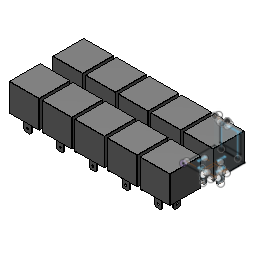
Блок реле с прозрачной крышкой т2 v2 (Autodesk Fusion 360 design; units mm, degrees)
Autodesk Fusion 360 part; units mm, degrees
sketch "Sketch1" plane through (0, 0, 0) normal (0, 0, 1) x (1, 0, 0)
  line L0 (0, 0) -> (27.5, 0)
  line L1 (27.5, 0) -> (27.5, 28.5)
  line L2 (27.5, 28.5) -> (0, 28.5)
  line L3 (0, 28.5) -> (0, 0)
  dimension "d1" = 27.5
  dimension "d2" = 28.5
  constraint horizontal L0
  constraint vertical L1
  constraint horizontal L2
  constraint vertical L3
  constraint coincident L0.start L3.end
  measures "d1" distance of L0.start L0.end
  measures "d2" distance of L0.start L2.end
extrude "Extrude1" add sketch "Sketch1" along normal blind 25.2 makes body 1
sketch "Sketch2" plane through (0, 0, 0) normal (0, 0, 1) x (1, 0, 0)
  line L0 (0, 3) -> (17, 3) construction
  line L1 (27.5, 4) -> (10.5, 4) construction
  line L2 (18, 0) -> (18, 4) construction
  line L3 (17, 4) -> (10.5, 4)
  line L4 (10.5, 4) -> (10.5, 3.1)
  line L5 (10.5, 3.1) -> (17, 3.1)
  line L6 (17, 3.1) -> (17, 4)
  line L7 (25, 0) -> (25, 15) construction
  line L8 (25, 15) -> (24, 15) construction
  line L9 (24, 15) -> (24, 8.7) construction
  line L10 (27.5, 12) -> (21.5, 12) construction
  line L11 (21.5, 8.7) -> (21.5, 15)
  line L12 (21.5, 15) -> (22.4, 15)
  line L13 (22.4, 15) -> (22.4, 8.7)
  line L14 (22.4, 8.7) -> (21.5, 8.7)
  line L15 (16, 4) -> (16, 18) construction
  line L16 (13.75, 4) -> (13.75, 18) construction
  line L17 (13.75, 18) -> (14.2, 18)
  line L18 (14.2, 18) -> (14.2, 24.3)
  line L19 (14.2, 24.3) -> (13.3, 24.3)
  line L20 (13.3, 24.3) -> (13.3, 18)
  line L21 (13.3, 18) -> (13.75, 18)
  line L22 (21.5, 13.8604) -> (5.5, 13.8604) construction
  line L23 (5.5, 15) -> (4.6, 15)
  line L24 (4.6, 15) -> (4.6, 8.7)
  line L25 (4.6, 8.7) -> (5.5, 8.7)
  line L26 (5.5, 8.7) -> (5.5, 15)
  dimension "d5" = 17
  dimension "d6" = 17
  dimension "d7" = 4
  dimension "d8" = 0.9
  dimension "d9" = 15
  dimension "d10" = 6.3
  dimension "d11" = 6
  dimension "d12" = 0.9
  dimension "d13" = 14
  dimension "d14" = 0.45
  dimension "d15" = 6.3
  dimension "d16" = 0.9
  dimension "d17" = 16
  dimension "d18" = 0.9
  constraint horizontal L0
  constraint horizontal L1
  constraint vertical L2
  constraint coincident L1 L3.start
  constraint perpendicular L2 L3
  constraint perpendicular L0 L4
  constraint perpendicular L4 L5
  constraint perpendicular L1 L7
  constraint perpendicular L7 L8
  constraint perpendicular L8 L9
  constraint parallel L3 L10
  constraint perpendicular L8 L11
  constraint perpendicular L11 L12
  constraint perpendicular L10 L13
  constraint perpendicular L11 L14
  constraint coincident L1 L15.start
  constraint perpendicular L1 L15
  constraint midpoint L3 L16.start
  constraint perpendicular L3 L16
  constraint perpendicular L16 L17
  constraint perpendicular L17 L18
  constraint perpendicular L18 L19
  constraint perpendicular L19 L20
  constraint perpendicular L16 L21
  constraint coincident L11 L22.start
  constraint perpendicular L16 L22
  constraint perpendicular L11 L23
  constraint perpendicular L14 L24
  constraint perpendicular L24 L25
  measures "d5" distance of L0.start L0.end
  measures "d6" distance of L1.start L1.end
  measures "d7" distance of L2.start L2.end
  measures "d8" distance of L1.end L4.end
  measures "d9" distance of L7.start L7.end
  measures "d10" distance of L8.end L9.end
  measures "d11" distance of L10.start L10.end
  measures "d12" distance of L11.end L12.end
  measures "d13" distance of L15.start L15.end
  measures "d14" distance of L16.end L17.end
  measures "d15" distance of L17.end L18.end
  measures "d16" distance of L18.end L19.end
  measures "d17" distance of L22.start L22.end
  measures "d18" distance of L23.start L23.end
extrude "Extrude2" add sketch "Sketch2" against normal blind 10.7 separate body makes body 2 at (5.5, 10.8, -7.1333) makes body 3 at (21.5, 10.8, -3.5667) makes body 4 at (14.8333, 4, -3.5667) makes body 5 at (13.3, 22.2, -3.5667)
chamfer "Chamfer1" distance 0.2 angle 45 8 edges at (5.5, 11.85, -10.7) (4.6, 11.85, -10.7) (21.5, 11.85, -10.7) (22.4, 11.85, -10.7) (13.75, 4, -10.7) (13.75, 3.1, -10.7) (14.2, 21.15, -10.7) (13.3, 21.15, -10.7) on bodies 2 3 4 5
chamfer "Chamfer4" distance 1.4 angle 45 8 edges at (5.05, 8.7, -10.7) (5.05, 15, -10.7) (21.95, 15, -10.7) (21.95, 8.7, -10.7) (17, 3.55, -10.7) (10.5, 3.55, -10.7) (13.75, 18, -10.7) (13.75, 24.3, -10.7) on bodies 2 3 4 5
sketch "Sketch3" plane through (0, 4, 0) normal (0, 1, 0) x (-1, 0, 0)
  line L0 (-11.7, -10.5) -> (-10.5, -9.3)
  line L1 (-10.5, -9.3) -> (-10.5, 0)
  line L2 (-10.5, 0) -> (-17, 0)
  line L3 (-17, 0) -> (-17, -9.3)
  line L4 (-17, -9.3) -> (-15.8, -10.5)
  line L5 (-15.8, -10.5) -> (-11.7, -10.5)
  line L6 (-13.75, -10.7045) -> (-13.75, -7.0045) construction
  circle A0 centre (-13.75, -7.0045) radius 0.9
  dimension "d25" = 3.7
  dimension "d26" = 1.8
  constraint perpendicular L5 L6
  constraint coincident L6.end A0.centre
  measures "d25" distance of L6.start L6.end
  measures "d26" diameter of A0
extrude "Extrude3" cut sketch "Sketch3" against normal blind 0.9 contours A0 bodies 4
sketch "Sketch4" plane through (5.5, 0, 0) normal (1, 0, 0) x (0, 1, 0)
  line L0 (13.8, -10.5) -> (15, -9.3)
  line L1 (15, -9.3) -> (15, 0)
  line L2 (15, 0) -> (8.7, 0)
  line L3 (8.7, 0) -> (8.7, -9.3)
  line L4 (8.7, -9.3) -> (9.9, -10.5)
  line L5 (9.9, -10.5) -> (13.8, -10.5)
  line L6 (11.85, -10.6992) -> (11.85, -6.9992) construction
  circle A0 centre (11.85, -6.9992) radius 0.9
  dimension "d29" = 3.7
  dimension "d30" = 1.8
  constraint perpendicular L5 L6
  constraint coincident L6.end A0.centre
  measures "d29" distance of L6.start L6.end
  measures "d30" diameter of A0
extrude "Extrude4" cut sketch "Sketch4" against normal blind 0.9 contours A0 bodies 2
sketch "Sketch5" plane through (22.4, 0, 0) normal (1, 0, 0) x (0, 1, 0)
  line L0 (8.7, -9.3) -> (9.9, -10.5)
  line L1 (9.9, -10.5) -> (13.8, -10.5)
  line L2 (13.8, -10.5) -> (15, -9.3)
  line L3 (15, -9.3) -> (15, 0)
  line L4 (15, 0) -> (8.7, 0)
  line L5 (8.7, 0) -> (8.7, -9.3)
  line L6 (11.85, -10.6965) -> (11.85, -6.9965) construction
  circle A0 centre (11.85, -6.9965) radius 0.9
  dimension "d33" = 3.7
  dimension "d34" = 1.8
  constraint perpendicular L1 L6
  constraint coincident L6.end A0.centre
  measures "d33" distance of L6.start L6.end
  measures "d34" diameter of A0
extrude "Extrude5" cut sketch "Sketch5" against normal blind 0.9 contours A0 bodies 3
sketch "Sketch6" plane through (14.2, 0, 0) normal (1, 0, 0) x (0, 1, 0)
  line L0 (23.1, -10.5) -> (24.3, -9.3)
  line L1 (24.3, -9.3) -> (24.3, 0)
  line L2 (24.3, 0) -> (18, 0)
  line L3 (18, 0) -> (18, -9.3)
  line L4 (18, -9.3) -> (19.2, -10.5)
  line L5 (19.2, -10.5) -> (23.1, -10.5)
  line L6 (21.15, -10.6998) -> (21.15, -6.9998) construction
  circle A0 centre (21.15, -6.9998) radius 0.9
  dimension "d37" = 3.7
  dimension "d38" = 1.8
  constraint perpendicular L5 L6
  constraint coincident L6.end A0.centre
  measures "d37" distance of L6.start L6.end
  measures "d38" diameter of A0
extrude "Extrude6" cut sketch "Sketch6" against normal blind 0.9 contours A0 bodies 5
fillet "Fillet1" radius 0.2 8 edges at (0, 0, 12.6) (27.5, 0, 12.6) (13.75, 0, 25.2) (27.5, 14.25, 25.2) (0, 14.25, 25.2) (13.75, 28.5, 25.2) (0, 28.5, 12.6) (27.5, 28.5, 12.6) on bodies 1
sketch "Sketch8" plane through (0, 28.5, 0) normal (0, 1, 0) x (-1, 0, 0)
  line L0 (-27.3, 25) -> (-27.3, 0)
  line L1 (-27.3, 0) -> (-0.2, 0)
  line L2 (-0.2, 0) -> (-0.2, 25)
  line L3 (-0.2, 25) -> (-27.3, 25)
  line L4 (-0.2, 23.5181) -> (-13.75, 23.5181) construction
  line L5 (-11.713, 25) -> (-11.713, 21.2) construction
  line L6 (-13.75, 21.2) -> (-6.25, 21.2)
  line L7 (-6.25, 21.2) -> (-6.25, 0)
  line L8 (-6.25, 0) -> (-21.25, 0)
  line L9 (-21.25, 21.2) -> (-21.25, 0)
  line L10 (-21.25, 21.2) -> (-13.75, 21.2)
  dimension "d46" = 13.55
  dimension "d47" = 3.8
  dimension "d48" = 7.5
  dimension "d49" = 15
  constraint coincident L2 L4.start
  constraint perpendicular L2 L4
  constraint coincident L3 L5.start
  constraint perpendicular L4 L5
  constraint perpendicular L5 L6
  constraint coincident L1 L7.end
  constraint perpendicular L1 L7
  constraint coincident L1 L8.end
  constraint perpendicular L8 L9
  constraint perpendicular L9 L10
  measures "d46" distance of L4.start L4.end
  measures "d47" distance of L5.start L5.end
  measures "d48" distance of L6.start L6.end
  measures "d49" distance of L7.end L8.end
sketch "Sketch9" plane through (0, 29.4, 0) normal (0, 1, 0) x (-1, 0, 0)
  line L0 (-21.25, 21.2) -> (-21.25, 0)
  line L1 (-21.25, 0) -> (-6.25, 0)
  line L2 (-6.25, 0) -> (-6.25, 21.2)
  line L3 (-6.25, 21.2) -> (-21.25, 21.2)
  line L4 (-6.25, 0) -> (-4.25, 0) construction
  line L5 (-4.25, 0) -> (-4.25, 4) construction
  line L6 (-3, 25) -> (-3, 21.2) construction
  line L7 (-6.25, 20.0587) -> (-4.25, 20.0587) construction
  line L8 (-4.25, 4) -> (-4.25, 21.2)
  line L9 (-4.25, 21.2) -> (-23.25, 21.2)
  line L10 (-23.25, 21.2) -> (-23.25, 4)
  line L11 (-23.25, 4) -> (-4.25, 4)
  dimension "d52" = 2
  dimension "d53" = 4
  dimension "d54" = 2
  dimension "d55" = 19
  constraint coincident L1.end L2.start
  constraint perpendicular L2 L4
  constraint perpendicular L4 L5
  constraint perpendicular L3 L6
  constraint coincident L2 L7.start
  constraint perpendicular L2 L7
  constraint perpendicular L7 L8
  constraint perpendicular L0 L9
  constraint perpendicular L9 L10
  constraint perpendicular L5 L11
  measures "d52" distance of L1.end L4.end
  measures "d53" distance of L4.end L5.end
  measures "d54" distance of L7.start L7.end
  measures "d55" distance of L8.end L9.end
extrude "Extrude8" add sketch "Sketch9" along normal blind 2.3 separate body contours L0 L2 L3 L9 L11 | L0 L9 L10 L11 | L2 L8 L9 L11 makes body 6
move_body "Move1" bodies 6 to x (1, 0, 0) y (0, 1, 0) z (0, 0, 1) at (0, -1, 0)
sketch "Sketch10" plane through (0, 0, 4) normal (0, 0, -1) x (1, 0, 0)
  line L0 (23.25, -28.4) -> (4.25, -28.4)
  line L1 (4.25, -28.4) -> (4.25, -30.7)
  line L2 (4.25, -30.7) -> (23.25, -30.7)
  line L3 (23.25, -30.7) -> (23.25, -28.4)
  line L4 (21.25, -28.5) -> (21.25, -29.4)
  line L5 (21.25, -29.4) -> (6.25, -29.4)
  line L6 (6.25, -29.4) -> (6.25, -28.5)
  line L7 (6.25, -28.5) -> (21.25, -28.5)
  constraint perpendicular L0 L4
  constraint perpendicular L4 L5
  constraint perpendicular L5 L6
  constraint perpendicular L4 L7
extrude "Extrude9" cut sketch "Sketch10" against normal blind 18 contours L4 L5 L6 L7 bodies 6
chamfer "Chamfer5" distance 0.6 angle 45 2 edges at (4.25, 30.7, 12.6) (23.25, 30.7, 12.6) on bodies 6
copy_body "CopyPasteBodies1" bodies 3 1 6 4 5 2 makes body 7 makes body 8 makes body 9 makes body 10 makes body 11 makes body 12
move_body "Move2" bodies 7 8 9 10 11 12 to x (1, 0, 0) y (0, 1, 0) z (0, 0, 1) at (-30, 0, 0)
copy_body "CopyPasteBodies2" bodies 3 1 6 4 5 2 makes body 13 makes body 14 makes body 15 makes body 16 makes body 17 makes body 18
move_body "Move3" bodies 13 14 15 16 17 18 to x (1, 0, 0) y (0, 1, 0) z (0, 0, 1) at (-60, 0, 0)
copy_body "CopyPasteBodies3" bodies 3 1 6 4 5 2 makes body 19 makes body 20 makes body 21 makes body 22 makes body 23 makes body 24
move_body "Move4" bodies 19 20 21 22 23 24 to x (1, 0, 0) y (0, 1, 0) z (0, 0, 1) at (-90, 0, 0)
copy_body "CopyPasteBodies4" bodies 3 1 6 4 5 2 makes body 25 makes body 26 makes body 27 makes body 28 makes body 29 makes body 30
move_body "Move5" bodies 25 26 27 28 29 30 to x (1, 0, 0) y (0, 1, 0) z (0, 0, 1) at (-120, 0, 0)
copy_body "CopyPasteBodies5" bodies 2 6 3 4 5 1 makes body 31 makes body 32 makes body 33 makes body 34 makes body 35 makes body 36
move_body "Move6" bodies 31 32 33 34 35 36 to x (1, 0, 0) y (0, 1, 0) z (0, 0, 1) at (0, -40, 0)
copy_body "CopyPasteBodies6" bodies 35 33 36 34 31 32 makes body 37 makes body 38 makes body 39 makes body 40 makes body 41 makes body 42
move_body "Move7" bodies 37 38 39 40 41 42 to x (1, 0, 0) y (0, 1, 0) z (0, 0, 1) at (-30, 0, 0)
copy_body "CopyPasteBodies7" bodies 41 42 38 32 31 37 35 34 39 40 36 33 makes body 43 makes body 44 makes body 45 makes body 46 makes body 47 makes body 48 makes body 49 makes body 50 makes body 51 makes body 52 makes body 53 makes body 54
move_body "Move8" bodies 43 44 45 46 47 48 49 50 51 52 53 54 to x (1, 0, 0) y (0, 1, 0) z (0, 0, 1) at (-60, 0, 0)
copy_body "CopyPasteBodies8" bodies 44 43 51 52 48 45 makes body 55 makes body 56 makes body 57 makes body 58 makes body 59 makes body 60
move_body "Move9" bodies 55 56 57 58 59 60 to x (1, 0, 0) y (0, 1, 0) z (0, 0, 1) at (-30, 0, 0)
